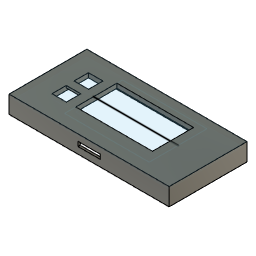
faceplate v7 (Autodesk Fusion 360 design; units mm, degrees)
Autodesk Fusion 360 part; units mm, degrees
note: some values were not read from the file. Chosen so that the rebuilt part matches the saved one: which face or edge a step refers to.
sketch "Sketch1" plane through (0, 0, 0) normal (0, 0, 1) x (1, 0, 0)
  line L0 (0, 0) -> (72, 0)
  line L1 (72, 0) -> (72, 35)
  line L2 (72, 35) -> (0, 35)
  line L3 (0, 35) -> (0, 0)
  dimension "d1" = 72
  dimension "d2" = 35
  constraint horizontal L0
  constraint vertical L1
  constraint horizontal L2
  constraint vertical L3
  constraint coincident L0.start L3.end
  measures "d1" distance of L0.start L0.end
  measures "d2" distance of L0.start L2.end
extrude "Extrude1" add sketch "Sketch1" along normal blind 1
extrude "Extrude2" add 1 faces at (24, 23.3333, 1) along direction (0, 0, 1) blind 2
sketch "Sketch2" plane through (0, 0, 3) normal (0, 0, 1) x (-1, 0, 0)
  line L0 (0, -35) -> (0, 0)
  line L1 (0, 0) -> (-72, 0)
  line L2 (-72, 0) -> (-72, -35)
  line L3 (-72, -35) -> (0, -35)
  line L4 (0, -21) -> (-16, -21)
  line L5 (-16, -21) -> (-5, -21)
  line L6 (-5, -21) -> (-5, -5)
  line L7 (-5, -5) -> (-16, -5)
  line L8 (-16, -5) -> (-16, -21)
  line L9 (-16, -21) -> (-5, -21)
  line L10 (-5, -21) -> (-5, -31)
  line L11 (-5, -31) -> (-16, -31)
  line L12 (-16, -31) -> (-16, -21)
  line L13 (-18, -31) -> (-58, -31)
  line L14 (-58, -31) -> (-58, -5)
  line L15 (-58, -5) -> (-18, -5)
  line L16 (-18, -5) -> (-18, -31)
  dimension "d7" = 16
  constraint coincident L0 L4.start
  constraint perpendicular L0 L4
  constraint horizontal L5
  constraint vertical L6
  constraint horizontal L7
  constraint vertical L8
  constraint horizontal L9
  constraint vertical L10
  constraint horizontal L11
  constraint vertical L12
  constraint horizontal L13
  constraint vertical L14
  constraint horizontal L15
  constraint vertical L16
  measures "d7" distance of L4.start L4.end
extrude "Extrude3" cut sketch "Sketch2" against normal blind 2 contours L4 L5 L9 L10 L11 L12 | L4 L5 L6 L7 L8 L9 | L13 L14 L15 L16
extrude "Extrude4" cut 1 faces at (24, 23.3333, 0) along direction (0, 0, 1) blind 1
sketch "Sketch3" plane through (0, 0, 1) normal (0, 0, -1) x (1, 0, 0)
  line L0 (58, -5) -> (58, -31)
  line L1 (58, -31) -> (18, -31)
  line L2 (18, -31) -> (18, -5)
  line L3 (18, -5) -> (58, -5)
  line L4 (5, -5) -> (16, -5)
  line L5 (16, -5) -> (16, -31)
  line L6 (16, -31) -> (5, -31)
  line L7 (5, -31) -> (5, -5)
  line L8 (0, 0) -> (0, -35)
  line L9 (0, -35) -> (72, -35)
  line L10 (72, -35) -> (72, 0)
  line L11 (72, 0) -> (0, 0)
  line L12 (70.5, 0) -> (70.5, -1)
  line L13 (70.5, -1) -> (0, -1)
  line L14 (70.5, -1) -> (72, -1)
  line L15 (72, -1) -> (71, -1)
  line L16 (71, -1) -> (71, -35)
  line L17 (72, -35) -> (72, -34)
  line L18 (72, -34) -> (0, -34)
  line L19 (0, -35) -> (1, -35)
  line L20 (1, -35) -> (1, 0)
  line L21 (0, 0) -> (72, 0)
  line L22 (72, 0) -> (72, -35)
  line L23 (72, -35) -> (0, -35)
  line L24 (0, -35) -> (0, 0)
  dimension "d12" = 1
  dimension "d13" = 1
  dimension "d14" = 1
  dimension "d15" = 72
  dimension "d16" = 1
  dimension "d17" = 35
  constraint coincident L11 L12.start
  constraint perpendicular L11 L12
  constraint coincident L8 L13.end
  constraint perpendicular L8 L13
  constraint coincident L10 L14.end
  constraint perpendicular L10 L14
  constraint perpendicular L10 L15
  constraint coincident L9 L16.end
  constraint perpendicular L9 L16
  constraint coincident L9.end L10.start
  constraint perpendicular L9 L17
  constraint perpendicular L8 L18
  constraint coincident L8.end L9.start
  constraint perpendicular L8 L19
  constraint perpendicular L11 L20
  constraint horizontal L21
  constraint vertical L22
  constraint horizontal L23
  constraint vertical L24
  constraint coincident L8.start L11.end
  measures "d12" distance of L12.start L12.end
  measures "d13" distance of L14.end L15.end
  measures "d14" distance of L9.end L17.end
  measures "d15" distance of L17.end L18.end
  measures "d16" distance of L8.end L19.end
  measures "d17" distance of L19.end L20.end
extrude "Extrude5" add sketch "Sketch3" along normal blind 5.9 contours L8 L11 L13 L20 L21 L24 | L8 L13 L18 L20 L24 | L11 L12 L13 L20 L21 | L8 L9 L18 L19 L20 L23 L24 | L10 L11 L12 L14 L15 L21 L22 | L9 L16 L18 L20 L23 | L9 L10 L16 L17 L18 L22 L23 | L10 L14 L15 L16 L18 L22
extrude "Extrude6" add 1 faces at (5, 13.6667, 2.3333) along direction (1, 0, 0) blind 4.5
sketch "Sketch4" plane through (0, 0, 3) normal (0, 0, 1) x (-1, 0, 0)
  line L0 (-58, -31) -> (-58, -5)
  line L1 (-58, -5) -> (-18, -5)
  line L2 (-18, -5) -> (-18, -31)
  line L3 (-18, -31) -> (-58, -31)
  line L4 (-16, -5) -> (-9.5, -5)
  line L5 (-9.5, -5) -> (-9.5, -31)
  line L6 (-9.5, -31) -> (-16, -31)
  line L7 (-16, -31) -> (-16, -5)
  line L8 (0, -35) -> (0, 0)
  line L9 (0, 0) -> (-72, 0)
  line L10 (-72, 0) -> (-72, -35)
  line L11 (-72, -35) -> (0, -35)
  line L12 (-16, -31) -> (-16, -18)
  line L13 (-16, -18) -> (-16, -16.25)
  line L14 (-16, -16.25) -> (-9.5, -16.25)
  line L15 (-9.5, -16.25) -> (-9.5, -19.75)
  line L16 (-9.5, -19.75) -> (-16, -19.7839)
  line L17 (-16, -19.7839) -> (-16, -16.25)
  dimension "d22" = 1.75
  dimension "d23" = 3.5
  constraint coincident L6.end L7.start
  constraint midpoint L7 L12.end
  constraint parallel L7 L13
  constraint coincident L5 L14.end
  constraint perpendicular L5 L14
  constraint perpendicular L14 L15
  constraint coincident L12 L16.end
  measures "d22" distance of L12.end L13.end
  measures "d23" distance of L14.end L15.end
extrude "Extrude7" add sketch "Sketch4" against normal blind 2 contours L5 L7 L12 L13 L14 L15 L16 L17
extrude "Extrude8" add 1 faces at (11.6667, 31, 2.3333) along direction (0, -1, 0) blind 4.8
extrude "Extrude9" add 1 faces at (11.6667, 5, 2.3333) along direction (0, 1, 0) blind 4.8
extrude "Extrude10" add 1 faces at (18, 13.6667, 2.3333) along direction (1, 0, 0) blind 2
sketch "Sketch5" plane through (0, 0, 3) normal (0, 0, 1) x (-1, 0, 0)
  line L0 (-16, -26.2) -> (-16, -19.7839)
  line L1 (-16, -19.7839) -> (-9.5, -19.75)
  line L2 (-9.5, -19.75) -> (-9.5, -26.2)
  line L3 (-9.5, -26.2) -> (-16, -26.2)
  line L4 (-58, -31) -> (-58, -5)
  line L5 (-58, -5) -> (-20, -5)
  line L6 (-20, -5) -> (-20, -31)
  line L7 (-20, -31) -> (-58, -31)
  line L8 (-9.5, -16.25) -> (-16, -16.25)
  line L9 (-16, -16.25) -> (-16, -9.8)
  line L10 (-16, -9.8) -> (-9.5, -9.8)
  line L11 (-9.5, -9.8) -> (-9.5, -16.25)
  line L12 (0, -35) -> (0, 0)
  line L13 (0, 0) -> (-72, 0)
  line L14 (-72, 0) -> (-72, -35)
  line L15 (-72, -35) -> (0, -35)
  line L16 (-20, -18) -> (-58, -18)
  constraint midpoint L6 L16.start
  constraint midpoint L4 L16.end
extrude "Extrude11" add 1 faces at (58, 22.3333, 2.3333) along direction (-1, 0, 0) blind 3.5
extrude "Extrude12" add 1 faces at (43, 5, 2.3333) along direction (0, 1, 0) blind 5
extrude "Extrude13" add 1 faces at (31.5, 31, 2.3333) along direction (0, -1, 0) blind 2.5
sketch "Sketch6" plane through (0, 0, 3) normal (0, 0, 1) x (-1, 0, 0)
sketch "Sketch7" plane through (0, 0, 1) normal (0, 0, -1) x (1, 0, 0)
  line L0 (16, -9.8) -> (16, -16.25)
  line L1 (16, -16.25) -> (9.5, -16.25)
  line L2 (9.5, -16.25) -> (9.5, -9.8)
  line L3 (9.5, -9.8) -> (16, -9.8)
  line L4 (1, -1) -> (1, -34)
  line L5 (1, -34) -> (71, -34)
  line L6 (71, -34) -> (71, -1)
  line L7 (71, -1) -> (1, -1)
  line L8 (20, -28.5) -> (20, -10)
  line L9 (20, -10) -> (54.5, -10)
  line L10 (54.5, -10) -> (54.5, -28.5)
  line L11 (54.5, -28.5) -> (20, -28.5)
  line L12 (9.5, -19.75) -> (16, -19.7839)
  line L13 (16, -19.7839) -> (16, -26.2)
  line L14 (16, -26.2) -> (9.5, -26.2)
  line L15 (9.5, -26.2) -> (9.5, -19.75)
sketch "Sketch8" plane through (0, 0, 3) normal (0, 0, 1) x (1, 0, 0)
  circle A0 centre (8.25, 29.75) radius 1.3
  circle A1 centre (8.25, 6.75) radius 1.3
  circle A2 centre (60.95, 29.75) radius 1.3
  circle A3 centre (60.95, 6.75) radius 1.3
  dimension "d45" = 2.6
  dimension "d46" = 2.6
  dimension "d47" = 2.6
  dimension "d48" = 2.6
  measures "d45" diameter of A0
  measures "d46" diameter of A1
  measures "d47" diameter of A2
  measures "d48" diameter of A3
sketch "Sketch11" plane through (0, 0, 1) normal (0, 0, -1) x (1, 0, 0)
  line L0 (0, -35) -> (8.5, -35)
  circle A0 centre (8.5, -29.2) radius 1.35
  circle A1 centre (8.5, -6.3) radius 1.35
  circle A2 centre (66.2, -6.3) radius 1.35
  circle A3 centre (66.2, -29.2) radius 1.35
  circle A4 centre (8.5, -6.3) radius 2
  circle A5 centre (8.5, -29.2) radius 2
  circle A6 centre (66.2, -6.3) radius 2
  circle A7 centre (66.2, -29.2) radius 2
  dimension "d66" = 5.8
  dimension "d67" = 2.7
  dimension "d68" = 22.9
  dimension "d69" = 2.7
  dimension "d70" = 57.7
  dimension "d71" = 2.7
  dimension "d72" = 22.9
  dimension "d73" = 2.7
  dimension "d74" = 4
  dimension "d75" = 4
  dimension "d76" = 4
  dimension "d77" = 4
  constraint horizontal L0
  measures "d66" distance of L0.end A0.centre
  measures "d67" diameter of A0
  measures "d68" distance of A0.centre A1.centre
  measures "d69" diameter of A1
  measures "d70" distance of A1.centre A2.centre
  measures "d71" diameter of A2
  measures "d72" distance of A2.centre A3.centre
  measures "d73" diameter of A3
  measures "d74" diameter of A4
  measures "d75" diameter of A5
  measures "d76" diameter of A6
  measures "d77" diameter of A7
extrude "Extrude17" add sketch "Sketch11" along normal blind 1.4
sketch "Sketch12" plane through (0, 0, -0.4) normal (0, 0, -1) x (1, 0, 0)
  circle A0 centre (66.2, -6.3) radius 1.35
  circle A1 centre (66.2, -6.3) radius 2
  circle A2 centre (66.2, -6.3) radius 1.35
  constraint concentric A0 A2
extrude "Extrude26" cut 4 faces at (64.7887, 30.2825, -0.4) (10.2709, 29.3664, -0.4) (10.2709, 6.4664, -0.4) (64.7887, 7.3825, -0.4) along direction (0, 0, 1) blind 1.3
extrude "Extrude27" add 4 faces at (64.7887, 30.2825, 0.9) (10.2709, 29.3664, 0.9) (10.2709, 6.4664, 0.9) (64.7887, 7.3825, 0.9) along direction (0, 0, 1) blind 0.1
sketch "Sketch21" plane through (0, 0, 1) normal (0, 0, -1) x (1, 0, 0)
  line L0 (9.5, -16.25) -> (16, -16.25)
  line L1 (16, -16.25) -> (16, -19.785)
  line L2 (16, -19.785) -> (9.5, -19.785)
  line L3 (9.5, -19.785) -> (9.5, -16.25)
  constraint horizontal L0
  constraint vertical L1
  constraint horizontal L2
  constraint vertical L3
extrude "Extrude28" cut sketch "Sketch21" against normal blind 1
sketch "Sketch22" plane through (0, 1, 0) normal (0, 1, 0) x (-1, 0, 0)
  line L0 (-1, 1) -> (-71, 1)
  line L1 (-71, 1) -> (-71, -4.9)
  line L2 (-71, -4.9) -> (-1, -4.9)
  line L3 (-1, -4.9) -> (-1, 1)
  line L4 (-71, 1) -> (-41, 1)
  line L5 (-71, -4.9) -> (-41, -4.9)
  line L6 (-41, -4.9) -> (-41, 0.1)
  line L7 (-41, 0.1) -> (-31, 0.1)
  line L8 (-31, 0.1) -> (-31, -1.9)
  line L9 (-31, -1.9) -> (-41, -1.9)
  line L10 (-41, -1.9) -> (-41, 0.1)
  dimension "d115" = 30
  dimension "d116" = 30
  dimension "d117" = 5
  dimension "d118" = 10
  dimension "d119" = 2
  constraint coincident L0.end L1.start
  constraint perpendicular L1 L4
  constraint coincident L1.end L2.start
  constraint perpendicular L1 L5
  constraint perpendicular L5 L6
  constraint horizontal L7
  constraint vertical L8
  constraint horizontal L9
  constraint vertical L10
  measures "d115" distance of L0.end L4.end
  measures "d116" distance of L1.end L5.end
  measures "d117" distance of L5.end L6.end
  measures "d118" distance of L6.end L7.end
  measures "d119" distance of L6.end L9.end
extrude "Extrude29" cut sketch "Sketch22" against normal blind 1 contours L6 L7 L8 L9 L10
sketch "Sketch23" plane through (0, 34, 0) normal (0, -1, 0) x (1, 0, 0)
  line L0 (71, 1) -> (1, 1)
  line L1 (1, 1) -> (1, -4.9)
  line L2 (1, -4.9) -> (71, -4.9)
  line L3 (71, -4.9) -> (71, 1)
  line L4 (1, -4.9) -> (31, -4.9)
  line L5 (31, -4.9) -> (31, 0.1)
  line L6 (31, 0.1) -> (41, 0.1)
  line L7 (41, 0.1) -> (41, -1.9)
  line L8 (41, -1.9) -> (31, -1.9)
  line L9 (31, -1.9) -> (31, 0.1)
  dimension "d122" = 30
  dimension "d123" = 5
  dimension "d124" = 10
  dimension "d125" = 2
  constraint coincident L1.end L2.start
  constraint perpendicular L3 L4
  constraint perpendicular L2 L5
  constraint horizontal L6
  constraint vertical L7
  constraint horizontal L8
  constraint vertical L9
  measures "d122" distance of L1.end L4.end
  measures "d123" distance of L4.end L5.end
  measures "d124" distance of L5.end L6.end
  measures "d125" distance of L5.end L8.end
extrude "Extrude30" cut sketch "Sketch23" against normal blind 1 contours L5 L6 L7 L8 L9
extrude "Extrude31" add 1 faces at (64.7887, 30.2825, 0.9) along direction (0, 0, 1) blind 0.1
extrude "Extrude18" [rolled back] along distance -10 taper angle 0
sketch "Sketch13" plane through (0, 0, -0.4) normal (0, 0, -1) x (1, 0, 0)
  circle A0 centre (8.5, -6.3) radius 1.35
  circle A1 centre (8.5, -6.3) radius 2
  circle A2 centre (8.5, -6.3) radius 1.35
  dimension "d82" = 2.7
  constraint concentric A0 A2
  measures "d82" diameter of A2
extrude "Extrude19" [rolled back] along distance -10 taper angle 0
sketch "Sketch14" plane through (0, 0, -0.4) normal (0, 0, -1) x (1, 0, 0)
  circle A0 centre (8.5, -29.2) radius 1.35
  circle A1 centre (8.5, -29.2) radius 2
  circle A2 centre (8.5, -29.2) radius 1.35
  dimension "d85" = 2.7
  constraint concentric A0 A2
  measures "d85" diameter of A2
extrude "Extrude20" [rolled back] along distance -10 taper angle 0
sketch "Sketch15" plane through (0, 0, -0.4) normal (0, 0, -1) x (1, 0, 0)
  circle A0 centre (66.2, -29.2) radius 1.35
  circle A1 centre (66.2, -29.2) radius 2
  circle A2 centre (66.2, -29.2) radius 1.35
  dimension "d88" = 2.7
  constraint concentric A0 A2
  measures "d88" diameter of A2
extrude "Extrude21" [rolled back] along distance -10 taper angle 0
fillet "Fillet2" [rolled back] radius 1
sketch "Sketch16" plane through (0, 0, -0.4) normal (0, 0, -1) x (1, 0, 0)
  circle A0 centre (66.2, -29.2) radius 1.35
  circle A1 centre (66.2, -29.2) radius 2
  circle A2 centre (66.2, -29.2) radius 1.5
  circle A3 centre (66.2, -29.2) radius 1.35
  dimension "d93" = 3
  dimension "d94" = 2.7
  constraint concentric A0 A2
  constraint concentric A2 A3
  measures "d93" diameter of A2
  measures "d94" diameter of A3
extrude "Extrude22" [rolled back] along distance -10 taper angle 0
sketch "Sketch17" plane through (0, 0, -0.4) normal (0, 0, -1) x (1, 0, 0)
  circle A0 centre (66.2, -6.3) radius 1.35
  circle A1 centre (66.2, -6.3) radius 2
  circle A2 centre (66.2, -6.3) radius 1.35
  circle A3 centre (66.2, -6.3) radius 1.5
  dimension "d97" = 2.7
  dimension "d98" = 3
  constraint concentric A0 A2
  constraint concentric A0 A3
  measures "d97" diameter of A2
  measures "d98" diameter of A3
extrude "Extrude23" [rolled back] along distance -10 taper angle 0
sketch "Sketch18" plane through (0, 0, -0.4) normal (0, 0, -1) x (1, 0, 0)
  circle A0 centre (8.5, -6.3) radius 1.35
  circle A1 centre (8.5, -6.3) radius 2
  circle A2 centre (8.5, -6.3) radius 1.35
  circle A3 centre (8.5, -6.3) radius 1.5
  dimension "d101" = 2.7
  dimension "d102" = 3
  constraint concentric A0 A2
  constraint concentric A0 A3
  measures "d101" diameter of A2
  measures "d102" diameter of A3
extrude "Extrude24" [rolled back] along distance -10 taper angle 0
sketch "Sketch19" plane through (0, 0, -0.4) normal (0, 0, -1) x (1, 0, 0)
  circle A0 centre (8.5, -29.2) radius 1.35
  circle A1 centre (8.5, -29.2) radius 2
  circle A2 centre (8.5, -29.2) radius 1.5
  circle A3 centre (8.5, -29.2) radius 1.35
  dimension "d105" = 3
  dimension "d106" = 2.7
  constraint concentric A0 A2
  constraint concentric A2 A3
  measures "d105" diameter of A2
  measures "d106" diameter of A3
extrude "Extrude25" [rolled back] along distance -10 taper angle 0
sketch "Sketch20" plane through (0, 0, 3) normal (0, 0, 1) x (-1, 0, 0)
